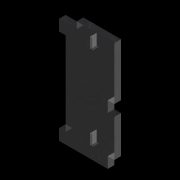
# Autodesk Inventor part: SideLeftLower
Saved by Autodesk Inventor 2019 (Build 230136000, 136)
## iProperties
Created: 2019-05-08
Part Number: SideLeftLower
Material: Acrylic, Clear
Document SubType Name: Modeling
Designer: super pig
Density: 1.19 g/cm^3
Appearance: Transparent - Clear
Mass: 3.5343 g
Surface Area: 25.305 cm^2
Volume: 2.97 cm^3
Name: Left Side Lower Cover
Author: super pig
Autodesk Inventor part; units mm, degrees
ref_plane "YZ Plane" through (0, 0, 0) normal (1, 0, 0) x (0, 1, 0)
ref_plane "XZ Plane" through (0, 0, 0) normal (0, 1, 0) x (-1, 0, 0)
ref_plane "XY Plane" through (0, 0, 0) normal (0, 0, 1) x (1, 0, 0)
sketch "Sketch1" plane through (0, 0, 0) normal (0, 0, 1) x (1, 0, 0)
  line L0 (-3, 4.65) -> (-3, 21.525)
  line L1 (0, 4.65) -> (-3, 4.65)
  line L2 (0, 21.525) -> (0, 4.65)
  line L3 (0, 21.525) -> (-3, 21.525)
  line L4 (-3, -0.35) -> (-3, 4.65)
  line L5 (-3, -0.35) -> (-22, -0.35)
  line L6 (-3, 21.525) -> (-3, 26.525)
  line L7 (-3, 26.525) -> (-3, 47.4)
  line L8 (0, 26.525) -> (-3, 26.525)
  line L9 (0, 47.4) -> (0, 26.525)
  line L10 (0, 47.4) -> (-3, 47.4)
  line L11 (-10, 47.4) -> (-10, 42.4)
  line L12 (-11, 47.4) -> (-10, 47.4)
  line L13 (-11, 42.4) -> (-11, 47.4)
  line L14 (-11, 42.4) -> (-10, 42.4)
  line L15 (-10, 9.65) -> (-10, 4.65)
  line L16 (-11, 9.65) -> (-10, 9.65)
  line L17 (-11, 4.65) -> (-11, 9.65)
  line L18 (-11, 4.65) -> (-10, 4.65)
  line L19 (0, 47.4) -> (0, 50.4)
  line L20 (0, 50.4) -> (-22, 50.4)
  line L21 (-22, 50.4) -> (-22, -0.35)
  line L22 (-22, -0.35) -> (-25, -0.35)
  line L23 (-25, -0.35) -> (-25, 4.65)
  line L24 (-25, 4.65) -> (-22, 4.65)
  line L25 (-22, 4.65) -> (-22, -0.35)
  line L26 (-22, 47.4) -> (-25, 47.4)
  line L27 (-25, 47.4) -> (-25, 42.4)
  line L28 (-25, 42.4) -> (-22, 42.4)
  line L29 (-22, 42.4) -> (-22, 47.4)
  line L30 (-22, 50.4) -> (-17, 50.4)
  line L31 (-17, 50.4) -> (-17, 47.4)
  line L32 (-17, 47.4) -> (-22, 47.4)
  line L33 (-22, 47.4) -> (-22, 50.4)
  line L34 (-25, -0.35) -> (-25, -5.35)
  point P0 (0, 0)
extrude "Extrusion1" add sketch "Sketch1" along normal blind 3 contours L4 L5 L21 L32 L31 L20 L19 L10 L7 L6 L0 | L0 L3 L2 L1 | L7 L10 L9 L8 | L22 L23 L24 L21 | L28 L27 L26 L21
body "Solid1"
